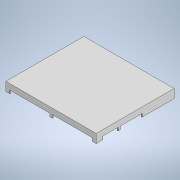
# Autodesk Inventor part: TopCase
Saved by Autodesk Inventor 2022 (Build 260153070, 153G)
## iProperties
Created: 2021-07-15
Part Number: TopCase
Material: Generic
Document SubType Name: Modeling
Designer: Eakawit_kor
Density: 1 g/cm^3
Appearance: Default
Author: Eakawit_kor
Autodesk Inventor part; units mm, degrees
ref_plane "YZ Plane" through (0, 0, 0) normal (1, 0, 0) x (0, 1, 0)
ref_plane "XZ Plane" through (0, 0, 0) normal (0, 1, 0) x (-1, 0, 0)
ref_plane "XY Plane" through (0, 0, 0) normal (0, 0, 1) x (1, 0, 0)
sketch "Sketch1" plane through (0, 0, 0) normal (0, 1, 0) x (-1, 0, 0)
  line L0 (0, 0) -> (102, 0)
  line L1 (102, 0) -> (102, -88)
  line L2 (102, -88) -> (0, -88)
  line L3 (0, -88) -> (0, 0)
  dimension "d0" = 102
  dimension "d1" = 88
  constraints: 8 end point, 2 parallel, 1 horizontal, 1 perpendicular
  measures "d0" distance of L0.start L0.end
  measures "d1" distance of L0.end L1.end
extrude "Extrusion1" add sketch "Sketch1" along normal blind 10
shell "Shell1" thickness 1 removed faces 1 at (-68, 0, -29.3333)
sketch "Sketch2" plane through (-102, 0, 0) normal (0, 0, 1) x (1, 0, 0)
  line L0 (1, 0) -> (101, 0) projected
  line L1 (4.398, 0) -> (49.698, 0)
  line L2 (49.698, 0) -> (49.698, 3.6)
  line L3 (49.698, 3.6) -> (4.398, 3.6)
  line L4 (4.398, 3.6) -> (4.398, 0)
  line L5 (52.298, 0) -> (97.598, 0)
  line L6 (97.598, 0) -> (97.598, 3.6)
  line L7 (97.598, 3.6) -> (52.298, 3.6)
  line L8 (52.298, 3.6) -> (52.298, 0)
  line L9 (101, 0) -> (101, 9) projected
  point P0 (102, 0)
  point P1 (49.698, 0)
  dimension "d5" = 45.3
  dimension "d6" = 2.6
  dimension "d7" = 3.402
  dimension "d8" = 3.6
  constraints: 16 end point, 4 parallel, 3 point on line, 2 horizontal, 2 perpendicular, 1 collinear
  measures "d5" distance of L2.end L3.end
  measures "d6" distance between parallel lines of L8 L2
  measures "d7" distance between parallel lines of L6 L9
  measures "d8" distance between parallel lines of L0 L7
extrude "Extrusion2" cut sketch "Sketch2" against normal up to surface (1 mm away)
sketch "Sketch3" plane through (0, 0, 0) normal (1, 0, 0) x (0, 0, -1)
  line L0 (7.371, 0) -> (24.671, 0)
  line L1 (24.671, 0) -> (24.671, 3.6)
  line L2 (24.671, 3.6) -> (7.371, 3.6)
  line L3 (7.371, 3.6) -> (7.371, 0)
  line L4 (88, 0) -> (0, 0) projected
  line L5 (27.5, 0) -> (51.8, 0)
  line L6 (51.8, 0) -> (51.8, 3.6)
  line L7 (51.8, 3.6) -> (27.5, 3.6)
  line L8 (27.5, 3.6) -> (27.5, 0)
  line L9 (0, 3.6) -> (0, 0) projected
  line L10 (1, 0) -> (1, 9) projected
  dimension "d12" = 6.371
  dimension "d13" = 17.3
  dimension "d15" = 2.829
  dimension "d16" = 24.3
  constraints: 16 end point, 6 parallel, 2 collinear, 2 horizontal, 2 perpendicular, 1 point on line
  measures "d12" distance between parallel lines of L10 L3
  measures "d13" distance of L1.end L2.end
  measures "d15" distance between parallel lines of L1 L8
  measures "d16" distance of L6.end L7.end
extrude "Extrusion3" cut sketch "Sketch3" against normal up to surface (1 mm away)
body "Solid1"
